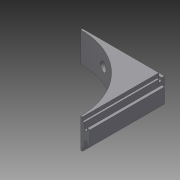
# Autodesk Inventor part: angolo-profilati
Saved by Autodesk Inventor 2014 SP1 (Build 180222100, 222)
## iProperties
Created: 2015-04-08
Part Number: angolo-profilati
Material: Generic
Document SubType Name: Modeling
Designer: Giorgio Nuzzo
Density: 1 g/cm^3
Appearance: Default
d5: 4,000 mm
d7: 4,000 mm
d17: 1,500 mm
d18: 40,000 mm
d19: 0,00 deg
d20: 1,500 mm
d21: 40,000 mm
d22: 0,00 deg
d23: 40,000 mm
d25: 0,00 deg
d26: 1,000 mm
d27: 5,000 mm
d28: 15,000 mm
d30: 0,00 deg
d31: 5,000 mm
d32: 10,000 mm
d34: 0,00 deg
Author: Giorgio Nuzzo
Autodesk Inventor part; units mm, degrees
ref_plane "Work Plane1" through (208, 234.75, 13.75) normal (0, 0, 1) x (1, 0, 0)
ref_plane "Work Plane2" through (180.5, 225, 24) normal (-1, 0, 0) x (0, -1, 0)
sketch "Sketch4" plane through (180.5, 225, 24) normal (-1, 0, 0) x (0, -1, 0)
  line L0 (-20.75, -21) -> (-18.75, -21) construction
  line L1 (-18.75, -21) -> (-18.75, -15.25) construction
  line L2 (-18.75, -15.25) -> (-24.5, -15.25) construction
  line L3 (-24.5, -15.25) -> (-24.5, -17.25) construction
  line L4 (-24.5, -17.25) -> (-25.5, -17.25) construction
  line L5 (-25.5, -17.25) -> (-25.5, -19.25) construction
  line L6 (-25.5, -19.25) -> (-26.5, -19.25) construction
  line L7 (-26.5, -19.25) -> (-26.5, -20.5) construction
  arc A0 (-26.5, -20.5) -> (-24, -23) centre (-24, -20.5) ccw construction
  line L8 (-24, -23) -> (-22.75, -23) construction
  line L9 (-22.75, -23) -> (-22.75, -22) construction
  line L10 (-22.75, -22) -> (-20.75, -22) construction
  line L11 (-20.75, -22) -> (-20.75, -21) construction
  line L12 (-24.5, -3.25) -> (-24.5, -5.25) construction
  line L13 (-24.5, -5.25) -> (-18.75, -5.25) construction
  line L14 (-18.75, -5.25) -> (-18.75, 0.5) construction
  line L15 (-18.75, 0.5) -> (-20.75, 0.5) construction
  line L16 (-20.75, 0.5) -> (-20.75, 1.5) construction
  line L17 (-20.75, 1.5) -> (-22.75, 1.5) construction
  line L18 (-22.75, 1.5) -> (-22.75, 2.5) construction
  line L19 (-22.75, 2.5) -> (-24, 2.5) construction
  arc A1 (-24, 2.5) -> (-26.5, 0) centre (-24, 0) ccw construction
  line L20 (-26.5, 0) -> (-26.5, -1.25) construction
  line L21 (-26.5, -1.25) -> (-25.5, -1.25) construction
  line L22 (-25.5, -1.25) -> (-25.5, -3.25) construction
  line L23 (-25.5, -3.25) -> (-24.5, -3.25) construction
  line L24 (-6.75, 0.5) -> (-8.75, 0.5) construction
  line L25 (-8.75, 0.5) -> (-8.75, -5.25) construction
  line L26 (-8.75, -5.25) -> (-3, -5.25) construction
  line L27 (-3, -5.25) -> (-3, -3.25) construction
  line L28 (-3, -3.25) -> (-2, -3.25) construction
  line L29 (-2, -3.25) -> (-2, -1.25) construction
  line L30 (-2, -1.25) -> (-1, -1.25) construction
  line L31 (-1, -1.25) -> (-1, 0) construction
  arc A2 (-1, 0) -> (-3.5, 2.5) centre (-3.5, 0) ccw construction
  line L32 (-3.5, 2.5) -> (-4.75, 2.5) construction
  line L33 (-4.75, 2.5) -> (-4.75, 1.5) construction
  line L34 (-4.75, 1.5) -> (-6.75, 1.5) construction
  line L35 (-6.75, 1.5) -> (-6.75, 0.5) construction
  line L36 (-3, -17.25) -> (-3, -15.25) construction
  line L37 (-3, -15.25) -> (-8.75, -15.25) construction
  line L38 (-8.75, -15.25) -> (-8.75, -21) construction
  line L39 (-8.75, -21) -> (-6.75, -21) construction
  line L40 (-6.75, -21) -> (-6.75, -22) construction
  line L41 (-6.75, -22) -> (-4.75, -22) construction
  line L42 (-4.75, -22) -> (-4.75, -23) construction
  line L43 (-4.75, -23) -> (-3.5, -23) construction
  arc A3 (-3.5, -23) -> (-1, -20.5) centre (-3.5, -20.5) ccw construction
  line L44 (-1, -20.5) -> (-1, -19.25) construction
  line L45 (-1, -19.25) -> (-2, -19.25) construction
  line L46 (-2, -19.25) -> (-2, -17.25) construction
  line L47 (-2, -17.25) -> (-3, -17.25) construction
  line L48 (-11.2751, -13.432) -> (-10.568, -12.7249) construction
  line L49 (-10.568, -12.7249) -> (-11.6644, -11.6285) construction
  arc A4 (-11.6644, -11.6285) -> (-11.6644, -8.8715) centre (-13.75, -10.25) ccw construction
  line L50 (-11.6644, -8.8715) -> (-10.568, -7.7751) construction
  line L51 (-10.568, -7.7751) -> (-11.2751, -7.068) construction
  line L52 (-11.2751, -7.068) -> (-12.3715, -8.1644) construction
  arc A5 (-12.3715, -8.1644) -> (-15.1285, -8.1644) centre (-13.75, -10.25) ccw construction
  line L53 (-15.1285, -8.1644) -> (-16.2249, -7.068) construction
  line L54 (-16.2249, -7.068) -> (-16.932, -7.7751) construction
  line L55 (-16.932, -7.7751) -> (-15.8356, -8.8715) construction
  arc A6 (-15.8356, -8.8715) -> (-15.8356, -11.6285) centre (-13.75, -10.25) ccw construction
  line L56 (-15.8356, -11.6285) -> (-16.932, -12.7249) construction
  line L57 (-16.932, -12.7249) -> (-16.2249, -13.432) construction
  line L58 (-16.2249, -13.432) -> (-15.1285, -12.3356) construction
  arc A7 (-15.1285, -12.3356) -> (-12.3715, -12.3356) centre (-13.75, -10.25) ccw construction
  line L59 (-12.3715, -12.3356) -> (-11.2751, -13.432) construction
  line L60 (-3.5, -14.25) -> (-3.5, -12.75) construction
  line L61 (-3.5, -12.75) -> (-2, -12.75) construction
  line L62 (-2, -12.75) -> (-2, -16.25) construction
  line L63 (-2, -16.25) -> (-1, -16.25) construction
  line L64 (-1, -16.25) -> (-1, -18.25) construction
  line L65 (-1, -18.25) -> (0, -18.25) construction
  line L66 (0, -18.25) -> (0, -20.5) construction
  arc A8 (-3.5, -24) -> (0, -20.5) centre (-3.5, -20.5) ccw construction
  line L67 (-3.5, -24) -> (-5.75, -24) construction
  line L68 (-5.75, -24) -> (-5.75, -23) construction
  line L69 (-5.75, -23) -> (-7.75, -23) construction
  line L70 (-7.75, -23) -> (-7.75, -22) construction
  line L71 (-7.75, -22) -> (-11.25, -22) construction
  line L72 (-11.25, -22) -> (-11.25, -20.5) construction
  line L73 (-11.25, -20.5) -> (-9.75, -20.5) construction
  line L74 (-9.75, -20.5) -> (-9.75, -15.25) construction
  line L75 (-9.75, -15.25) -> (-17.75, -15.25) construction
  line L76 (-17.75, -15.25) -> (-17.75, -20.5) construction
  line L77 (-17.75, -20.5) -> (-16.25, -20.5) construction
  line L78 (-16.25, -20.5) -> (-16.25, -22) construction
  line L79 (-16.25, -22) -> (-19.75, -22) construction
  line L80 (-19.75, -22) -> (-19.75, -23) construction
  line L81 (-19.75, -23) -> (-21.75, -23) construction
  line L82 (-21.75, -23) -> (-21.75, -24) construction
  line L83 (-21.75, -24) -> (-24, -24) construction
  arc A9 (-27.5, -20.5) -> (-24, -24) centre (-24, -20.5) ccw construction
  line L84 (-27.5, -20.5) -> (-27.5, -18.25) construction
  line L85 (-27.5, -18.25) -> (-26.5, -18.25) construction
  line L86 (-26.5, -18.25) -> (-26.5, -16.25) construction
  line L87 (-26.5, -16.25) -> (-25.5, -16.25) construction
  line L88 (-25.5, -16.25) -> (-25.5, -12.75) construction
  line L89 (-25.5, -12.75) -> (-24, -12.75) construction
  line L90 (-24, -12.75) -> (-24, -14.25) construction
  line L91 (-24, -14.25) -> (-18.75, -14.25) construction
  line L92 (-18.75, -14.25) -> (-18.75, -6.25) construction
  line L93 (-18.75, -6.25) -> (-24, -6.25) construction
  line L94 (-24, -6.25) -> (-24, -7.75) construction
  line L95 (-24, -7.75) -> (-25.5, -7.75) construction
  line L96 (-25.5, -7.75) -> (-25.5, -4.25) construction
  line L97 (-25.5, -4.25) -> (-26.5, -4.25) construction
  line L98 (-26.5, -4.25) -> (-26.5, -2.25) construction
  line L99 (-26.5, -2.25) -> (-27.5, -2.25) construction
  line L100 (-27.5, -2.25) -> (-27.5, 0) construction
  arc A10 (-24, 3.5) -> (-27.5, 0) centre (-24, 0) ccw construction
  line L101 (-24, 3.5) -> (-21.75, 3.5) construction
  line L102 (-21.75, 3.5) -> (-21.75, 2.5) construction
  line L103 (-21.75, 2.5) -> (-19.75, 2.5) construction
  line L104 (-19.75, 2.5) -> (-19.75, 1.5) construction
  line L105 (-19.75, 1.5) -> (-16.25, 1.5) construction
  line L106 (-16.25, 1.5) -> (-16.25, 0) construction
  line L107 (-16.25, 0) -> (-17.75, 0) construction
  line L108 (-17.75, 0) -> (-17.75, -5.25) construction
  line L109 (-17.75, -5.25) -> (-9.75, -5.25) construction
  line L110 (-9.75, -5.25) -> (-9.75, 0) construction
  line L111 (-9.75, 0) -> (-11.25, 0) construction
  line L112 (-11.25, 0) -> (-11.25, 1.5) construction
  line L113 (-11.25, 1.5) -> (-7.75, 1.5) construction
  line L114 (-7.75, 1.5) -> (-7.75, 2.5) construction
  line L115 (-7.75, 2.5) -> (-5.75, 2.5) construction
  line L116 (-5.75, 2.5) -> (-5.75, 3.5) construction
  line L117 (-5.75, 3.5) -> (-3.5, 3.5) construction
  arc A11 (0, 0) -> (-3.5, 3.5) centre (-3.5, 0) ccw construction
  line L118 (0, 0) -> (0, -2.25) construction
  line L119 (0, -2.25) -> (-1, -2.25) construction
  line L120 (-1, -2.25) -> (-1, -4.25) construction
  line L121 (-1, -4.25) -> (-2, -4.25) construction
  line L122 (-2, -4.25) -> (-2, -7.75) construction
  line L123 (-2, -7.75) -> (-3.5, -7.75) construction
  line L124 (-3.5, -7.75) -> (-3.5, -6.25) construction
  line L125 (-3.5, -6.25) -> (-8.75, -6.25) construction
  line L126 (-8.75, -6.25) -> (-8.75, -14.25) construction
  line L127 (-8.75, -14.25) -> (-3.5, -14.25) construction
  line L128 (-3.5, -12.75) -> (-3.5, -14.25)
  line L129 (-3.5, -14.25) -> (-5, -14.25)
  line L130 (-5, -14.25) -> (-5, -6.25)
  line L131 (-3.5, -6.25) -> (-5, -6.25)
  line L132 (-3.5, -6.25) -> (-3.5, -7.75)
  line L133 (-3.5, -7.75) -> (-2, -7.75)
  line L134 (-3.5, -12.75) -> (-2, -12.75)
  line L135 (-2, -16.25) -> (-2, -12.75)
  line L136 (-2, -16.25) -> (-1, -16.25)
  line L137 (-1, -18.25) -> (-1, -16.25)
  line L138 (-1, -18.25) -> (0, -18.25)
  line L139 (-2, -7.75) -> (-2, -4.25)
  line L140 (-1, -4.25) -> (-2, -4.25)
  line L141 (-1, -4.25) -> (-1, -2.25)
  line L142 (0, -2.25) -> (-1, -2.25)
  line L143 (0, -18.25) -> (0, -2.25)
  point P0 (225, -24)
  dimension "d17" = 1.5
  constraints: 288 end point, 58 horizontal, 58 vertical, 24 point on circle, 12 centre point, 10 perpendicular, 3 collinear, 2 parallel, 2 point on line, 176 other
  measures "d17" distance of L60.start L129.end
extrude "Extrusion4" add sketch "Sketch4" along normal blind 40
ref_plane "Work Plane3" through (208, 225, 3.5) normal (0, -1, 0) x (-1, 0, 0)
sketch "Sketch5" plane through (208, 225, 3.5) normal (0, -1, 0) x (-1, 0, 0)
  line L0 (6.75, -21) -> (8.75, -21) construction
  line L1 (8.75, -21) -> (8.75, -15.25) construction
  line L2 (8.75, -15.25) -> (3, -15.25) construction
  line L3 (3, -15.25) -> (3, -17.25) construction
  line L4 (3, -17.25) -> (2, -17.25) construction
  line L5 (2, -17.25) -> (2, -19.25) construction
  line L6 (2, -19.25) -> (1, -19.25) construction
  line L7 (1, -19.25) -> (1, -20.5) construction
  arc A0 (1, -20.5) -> (3.5, -23) centre (3.5, -20.5) ccw construction
  line L8 (3.5, -23) -> (4.75, -23) construction
  line L9 (4.75, -23) -> (4.75, -22) construction
  line L10 (4.75, -22) -> (6.75, -22) construction
  line L11 (6.75, -22) -> (6.75, -21) construction
  line L12 (3, -3.25) -> (3, -5.25) construction
  line L13 (3, -5.25) -> (8.75, -5.25) construction
  line L14 (8.75, -5.25) -> (8.75, 0.5) construction
  line L15 (8.75, 0.5) -> (6.75, 0.5) construction
  line L16 (6.75, 0.5) -> (6.75, 1.5) construction
  line L17 (6.75, 1.5) -> (4.75, 1.5) construction
  line L18 (4.75, 1.5) -> (4.75, 2.5) construction
  line L19 (4.75, 2.5) -> (3.5, 2.5) construction
  arc A1 (3.5, 2.5) -> (1, 0) centre (3.5, 0) ccw construction
  line L20 (1, 0) -> (1, -1.25) construction
  line L21 (1, -1.25) -> (2, -1.25) construction
  line L22 (2, -1.25) -> (2, -3.25) construction
  line L23 (2, -3.25) -> (3, -3.25) construction
  line L24 (20.75, 0.5) -> (18.75, 0.5) construction
  line L25 (18.75, 0.5) -> (18.75, -5.25) construction
  line L26 (18.75, -5.25) -> (24.5, -5.25) construction
  line L27 (24.5, -5.25) -> (24.5, -3.25) construction
  line L28 (24.5, -3.25) -> (25.5, -3.25) construction
  line L29 (25.5, -3.25) -> (25.5, -1.25) construction
  line L30 (25.5, -1.25) -> (26.5, -1.25) construction
  line L31 (26.5, -1.25) -> (26.5, 0) construction
  arc A2 (26.5, 0) -> (24, 2.5) centre (24, 0) ccw construction
  line L32 (24, 2.5) -> (22.75, 2.5) construction
  line L33 (22.75, 2.5) -> (22.75, 1.5) construction
  line L34 (22.75, 1.5) -> (20.75, 1.5) construction
  line L35 (20.75, 1.5) -> (20.75, 0.5) construction
  line L36 (24.5, -17.25) -> (24.5, -15.25) construction
  line L37 (24.5, -15.25) -> (18.75, -15.25) construction
  line L38 (18.75, -15.25) -> (18.75, -21) construction
  line L39 (18.75, -21) -> (20.75, -21) construction
  line L40 (20.75, -21) -> (20.75, -22) construction
  line L41 (20.75, -22) -> (22.75, -22) construction
  line L42 (22.75, -22) -> (22.75, -23) construction
  line L43 (22.75, -23) -> (24, -23) construction
  arc A3 (24, -23) -> (26.5, -20.5) centre (24, -20.5) ccw construction
  line L44 (26.5, -20.5) -> (26.5, -19.25) construction
  line L45 (26.5, -19.25) -> (25.5, -19.25) construction
  line L46 (25.5, -19.25) -> (25.5, -17.25) construction
  line L47 (25.5, -17.25) -> (24.5, -17.25) construction
  line L48 (16.2249, -13.432) -> (16.932, -12.7249) construction
  line L49 (16.932, -12.7249) -> (15.8356, -11.6285) construction
  arc A4 (15.8356, -11.6285) -> (15.8356, -8.8715) centre (13.75, -10.25) ccw construction
  line L50 (15.8356, -8.8715) -> (16.932, -7.7751) construction
  line L51 (16.932, -7.7751) -> (16.2249, -7.068) construction
  line L52 (16.2249, -7.068) -> (15.1285, -8.1644) construction
  arc A5 (15.1285, -8.1644) -> (12.3715, -8.1644) centre (13.75, -10.25) ccw construction
  line L53 (12.3715, -8.1644) -> (11.2751, -7.068) construction
  line L54 (11.2751, -7.068) -> (10.568, -7.7751) construction
  line L55 (10.568, -7.7751) -> (11.6644, -8.8715) construction
  arc A6 (11.6644, -8.8715) -> (11.6644, -11.6285) centre (13.75, -10.25) ccw construction
  line L56 (11.6644, -11.6285) -> (10.568, -12.7249) construction
  line L57 (10.568, -12.7249) -> (11.2751, -13.432) construction
  line L58 (11.2751, -13.432) -> (12.3715, -12.3356) construction
  arc A7 (12.3715, -12.3356) -> (15.1285, -12.3356) centre (13.75, -10.25) ccw construction
  line L59 (15.1285, -12.3356) -> (16.2249, -13.432) construction
  line L60 (24, -14.25) -> (24, -12.75) construction
  line L61 (24, -12.75) -> (25.5, -12.75) construction
  line L62 (25.5, -12.75) -> (25.5, -16.25) construction
  line L63 (25.5, -16.25) -> (26.5, -16.25) construction
  line L64 (26.5, -16.25) -> (26.5, -18.25) construction
  line L65 (26.5, -18.25) -> (27.5, -18.25) construction
  line L66 (27.5, -18.25) -> (27.5, -20.5) construction
  arc A8 (24, -24) -> (27.5, -20.5) centre (24, -20.5) ccw construction
  line L67 (24, -24) -> (21.75, -24) construction
  line L68 (21.75, -24) -> (21.75, -23) construction
  line L69 (21.75, -23) -> (19.75, -23) construction
  line L70 (19.75, -23) -> (19.75, -22) construction
  line L71 (19.75, -22) -> (16.25, -22) construction
  line L72 (16.25, -22) -> (16.25, -20.5) construction
  line L73 (16.25, -20.5) -> (17.75, -20.5) construction
  line L74 (17.75, -20.5) -> (17.75, -15.25) construction
  line L75 (17.75, -15.25) -> (9.75, -15.25) construction
  line L76 (9.75, -15.25) -> (9.75, -20.5) construction
  line L77 (9.75, -20.5) -> (11.25, -20.5) construction
  line L78 (11.25, -20.5) -> (11.25, -22) construction
  line L79 (11.25, -22) -> (7.75, -22) construction
  line L80 (7.75, -22) -> (7.75, -23) construction
  line L81 (7.75, -23) -> (5.75, -23) construction
  line L82 (5.75, -23) -> (5.75, -24) construction
  line L83 (5.75, -24) -> (3.5, -24) construction
  arc A9 (0, -20.5) -> (3.5, -24) centre (3.5, -20.5) ccw construction
  line L84 (0, -20.5) -> (0, -18.25) construction
  line L85 (0, -18.25) -> (1, -18.25) construction
  line L86 (1, -18.25) -> (1, -16.25) construction
  line L87 (1, -16.25) -> (2, -16.25) construction
  line L88 (2, -16.25) -> (2, -12.75) construction
  line L89 (2, -12.75) -> (3.5, -12.75) construction
  line L90 (3.5, -12.75) -> (3.5, -14.25) construction
  line L91 (3.5, -14.25) -> (8.75, -14.25) construction
  line L92 (8.75, -14.25) -> (8.75, -6.25) construction
  line L93 (8.75, -6.25) -> (3.5, -6.25) construction
  line L94 (3.5, -6.25) -> (3.5, -7.75) construction
  line L95 (3.5, -7.75) -> (2, -7.75) construction
  line L96 (2, -7.75) -> (2, -4.25) construction
  line L97 (2, -4.25) -> (1, -4.25) construction
  line L98 (1, -4.25) -> (1, -2.25) construction
  line L99 (1, -2.25) -> (0, -2.25) construction
  line L100 (0, -2.25) -> (0, 0) construction
  arc A10 (3.5, 3.5) -> (0, 0) centre (3.5, 0) ccw construction
  line L101 (3.5, 3.5) -> (5.75, 3.5) construction
  line L102 (5.75, 3.5) -> (5.75, 2.5) construction
  line L103 (5.75, 2.5) -> (7.75, 2.5) construction
  line L104 (7.75, 2.5) -> (7.75, 1.5) construction
  line L105 (7.75, 1.5) -> (11.25, 1.5) construction
  line L106 (11.25, 1.5) -> (11.25, 0) construction
  line L107 (11.25, 0) -> (9.75, 0) construction
  line L108 (9.75, 0) -> (9.75, -5.25) construction
  line L109 (9.75, -5.25) -> (17.75, -5.25) construction
  line L110 (17.75, -5.25) -> (17.75, 0) construction
  line L111 (17.75, 0) -> (16.25, 0) construction
  line L112 (16.25, 0) -> (16.25, 1.5) construction
  line L113 (16.25, 1.5) -> (19.75, 1.5) construction
  line L114 (19.75, 1.5) -> (19.75, 2.5) construction
  line L115 (19.75, 2.5) -> (21.75, 2.5) construction
  line L116 (21.75, 2.5) -> (21.75, 3.5) construction
  line L117 (21.75, 3.5) -> (24, 3.5) construction
  arc A11 (27.5, 0) -> (24, 3.5) centre (24, 0) ccw construction
  line L118 (27.5, 0) -> (27.5, -2.25) construction
  line L119 (27.5, -2.25) -> (26.5, -2.25) construction
  line L120 (26.5, -2.25) -> (26.5, -4.25) construction
  line L121 (26.5, -4.25) -> (25.5, -4.25) construction
  line L122 (25.5, -4.25) -> (25.5, -7.75) construction
  line L123 (25.5, -7.75) -> (24, -7.75) construction
  line L124 (24, -7.75) -> (24, -6.25) construction
  line L125 (24, -6.25) -> (18.75, -6.25) construction
  line L126 (18.75, -6.25) -> (18.75, -14.25) construction
  line L127 (18.75, -14.25) -> (24, -14.25) construction
  line L128 (27.5, -18.25) -> (26.5, -18.25)
  line L129 (26.5, -16.25) -> (26.5, -18.25)
  line L130 (26.5, -16.25) -> (25.5, -16.25)
  line L131 (25.5, -16.25) -> (25.5, -12.75)
  line L132 (24, -12.75) -> (25.5, -12.75)
  line L133 (24, -12.75) -> (24, -14.25)
  line L134 (24, -14.25) -> (22.5, -14.25)
  line L135 (22.5, -14.25) -> (22.5, -6.25)
  line L136 (24, -6.25) -> (22.5, -6.25)
  line L137 (24, -6.25) -> (24, -7.75)
  line L138 (25.5, -7.75) -> (24, -7.75)
  line L139 (25.5, -7.75) -> (25.5, -4.25)
  line L140 (25.5, -4.25) -> (26.5, -4.25)
  line L141 (26.5, -2.25) -> (26.5, -4.25)
  line L142 (26.5, -2.25) -> (27.5, -2.25)
  line L143 (27.5, -18.25) -> (27.5, -2.25)
  point P0 (208, 3.5)
  dimension "d20" = 1.5
  constraints: 288 end point, 58 horizontal, 58 vertical, 24 point on circle, 13 perpendicular, 12 centre point, 2 point on line, 1 collinear, 1 parallel, 176 other
  measures "d20" distance of L60.start L134.end
extrude "Extrusion5" add sketch "Sketch5" along normal blind 40
sketch "Sketch6" plane through (140.5, 226, 21.75) normal (0, 0, 1) x (1, 0, 0)
  line L0 (40, 0) -> (0, 0) construction
  line L1 (40, -1) -> (0, -1) construction
  line L2 (40, -1) -> (40, -41) construction
  arc A0 (40, -41) -> (0, -1) centre (0, -41) ccw
  line L3 (0, -1) -> (40, -1)
  line L4 (40, -41) -> (40, -1)
  line L5 (40, 0) -> (41, 0)
  line L6 (41, 0) -> (41, -1)
  line L7 (41, -1) -> (40, -1)
  line L8 (40, -1) -> (40, 0)
  point P0 (-140.5, -226)
  dimension "d23" = 40
  dimension "d26" = 1
  constraints: 14 end point, 4 equal length, 2 point on circle, 1 centre point, 1 horizontal, 1 perpendicular
  measures "d23" radius of A0
  measures "d26" distance of L6.end L7.end
extrude "Extrusion6" add sketch "Sketch6" against normal up to surface (16 mm away)
sketch "Sketch7" plane through (140.5, 226, 19.75) normal (0, 1, 0) x (1, 0, 0)
  line L0 (0, 12) -> (0, 14) projected
  circle A0 centre (15, 6) radius 2.5
  point P0 (-140.5, 19.75)
  dimension "d27" = 5
  dimension "d28" = 15
  constraints: 1 centre point
  measures "d27" diameter of A0
  measures "d28" distance from line of L0 A0.centre
extrude "Extrusion7" cut sketch "Sketch7" against normal through all
sketch "Sketch8" plane through (181.5, 185, 21.75) normal (1, 0, 0) x (0, 0, -1)
  line L0 (16, 0) -> (14, 0) projected
  circle A0 centre (8, 10) radius 2.5
  point P0 (21.75, -185)
  dimension "d31" = 5
  dimension "d32" = 10
  constraints: 1 centre point
  measures "d31" diameter of A0
  measures "d32" distance from line of L0 A0.centre
extrude "Extrusion8" cut sketch "Sketch8" against normal through all
equation "\"d7\" = d5"
equation "\"d5\" = 4"
body "Solid2"
